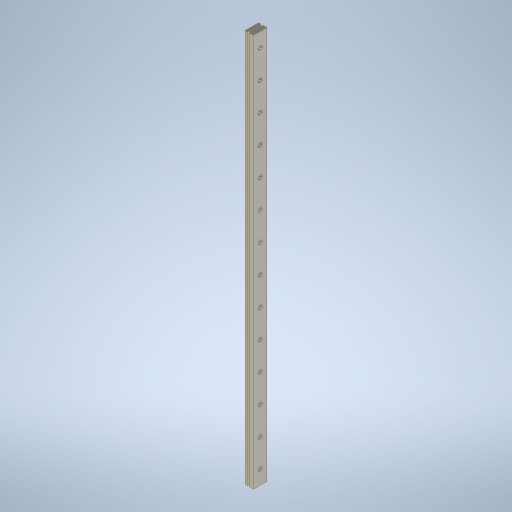
# Autodesk Inventor part: Trilho
Saved by Autodesk Inventor 2023 (Build 270158000, 158)
## iProperties
Created: 2023-03-17
Part Number: Trilho
Material: Aço inoxidável
Document SubType Name: Sheet Metal
Designer: Mateus
Density: 8 g/cm^3
Sheet Metal Rule: Default_mm
Appearance: Prata
Mass: 219.806 g
Surface Area: 172.742 cm^2
Volume: 27.4758 cm^3
Author: Mateus
Autodesk Inventor part; units mm, degrees
ref_plane "YZ Plane" through (0, 0, 0) normal (1, 0, 0) x (0, 1, 0)
ref_plane "XZ Plane" through (0, 0, 0) normal (0, 1, 0) x (-1, 0, 0)
ref_plane "XY Plane" through (0, 0, 0) normal (0, 0, 1) x (1, 0, 0)
sketch "Esboço1" plane through (0, 0, 0) normal (0, 1, 0) x (-1, 0, 0)
  line L0 (0, 0) -> (3.5, 0)
  line L1 (4, -2) -> (5, -2)
  line L2 (5.5, 0) -> (7.5, 0)
  line L3 (7.5, 0) -> (7.5, -12)
  line L4 (7.5, -12) -> (5.5, -12)
  line L5 (5, -10) -> (4, -10)
  line L6 (3.5, -12) -> (0, -12)
  line L7 (0, -12) -> (0, 0)
  line L8 (5.5, 0) -> (5, -2)
  line L9 (3.5, 0) -> (4, -2)
  line L10 (5, -10) -> (5.5, -12)
  line L11 (3.5, -12) -> (4, -10)
  dimension "d0" = 7.5
  dimension "d1" = 12
  dimension "d2" = 8
  dimension "d3" = 1
  dimension "d4" = 3.5
  dimension "d5" = 0.5
  constraints: 24 end point, 4 point on line, 3 equal length, 3 perpendicular, 1 horizontal, 1 parallel
  measures "d0" distance of L0.start L2.end
  measures "d1" distance of L6.end L0.start
  measures "d2" distance of L1.end L5.start
  measures "d3" distance of L1.start L1.end
  measures "d4" distance of L0.start L0.end
  measures "d5" horizontal distance of L2.start L1.end
extrude "Extrusão1" add sketch "Esboço1" along normal blind 350
sketch "Esboço2" plane through (-7.5, 0, -12) normal (-1, 0, 0) x (0, 0, 1)
  line L0 (0, 0) -> (12, 0) projected
  line L1 (12, 0) -> (12, 350) projected
  line L2 (0, 350) -> (12, 350) projected
  point P0 (6, 12.5)
  point P1 (6, 37.5)
  point P2 (6, 62.5)
  point P3 (6, 87.5)
  point P4 (6, 112.5)
  point P5 (6, 137.5)
  point P6 (6, 162.5)
  point P7 (6, 187.5)
  point P8 (6, 212.5)
  point P9 (6, 237.5)
  point P10 (6, 262.5)
  point P11 (6, 287.5)
  point P12 (6, 312.5)
  point P13 (6, 337.5)
  dimension "d8" = 25
  dimension "d9" = 12.5
  dimension "d10" = 12
  dimension "d11" = 6
  dimension "d12" = 6
  dimension "d13" = 25
  dimension "d14" = 25
  dimension "d15" = 25
  dimension "d16" = 25
  dimension "d17" = 25
  dimension "d18" = 25
  dimension "d19" = 25
  dimension "d20" = 25
  dimension "d21" = 25
  dimension "d22" = 25
  dimension "d23" = 25
  dimension "d24" = 25
  dimension "d25" = 12.5
  measures "d8" distance of point (6, 12.5) point (6, 37.5)
  measures "d9" distance from line of L0 point (6, 12.5)
  measures "d10" distance of L0.start L0.end
  measures "d11" distance from line of L1 point (6, 12.5)
  measures "d12" distance from line of L1 point (6, 287.5)
  measures "d13" distance of point (6, 62.5) point (6, 37.5)
  measures "d14" distance of point (6, 87.5) point (6, 62.5)
  measures "d15" distance of point (6, 112.5) point (6, 87.5)
  measures "d16" distance of point (6, 137.5) point (6, 112.5)
  measures "d17" distance of point (6, 137.5) point (6, 162.5)
  measures "d18" distance of point (6, 162.5) point (6, 187.5)
  measures "d19" distance of point (6, 187.5) point (6, 212.5)
  measures "d20" distance of point (6, 237.5) point (6, 212.5)
  measures "d21" distance of point (6, 237.5) point (6, 262.5)
  measures "d22" distance of point (6, 287.5) point (6, 262.5)
  measures "d23" distance of point (6, 287.5) point (6, 312.5)
  measures "d24" distance of point (6, 312.5) point (6, 337.5)
  measures "d25" distance from line of L2 point (6, 337.5)
hole "Furo1" at (-7.5, 12.5, -6) at (-7.5, 37.5, -6) at (-7.5, 62.5, -6) at (-7.5, 87.5, -6) at (-7.5, 112.5, -6) at (-7.5, 137.5, -6) at (-7.5, 162.5, -6) at (-7.5, 187.5, -6) at (-7.5, 212.5, -6) at (-7.5, 237.5, -6) at (-7.5, 262.5, -6) at (-7.5, 287.5, -6) at (-7.5, 312.5, -6) at (-7.5, 337.5, -6) direction (1, 0, 0) diameter 3.5 depth 7.5 counterbore diameter 6 counterbore depth 3.5
equation "\"d11\" = 0.5 * d10"
equation "\"d13\" = d8"
equation "\"d14\" = d13"
equation "\"d15\" = d13"
equation "\"d16\" = d14"
equation "\"d17\" = d16"
equation "\"d18\" = d17"
equation "\"d19\" = d17"
equation "\"d20\" = d18"
equation "\"d21\" = d19"
equation "\"d22\" = d20"
equation "\"d23\" = d21"
equation "\"d24\" = d22"
equation "\"d31\" = Espessura"
equation "\"Raio_vergadura\" = Espessura"
equation "\"Largura_alívio_de_vergadura\" = Espessura"
equation "\"Profundidade_alívio_de_vergadura\" = 0.5 * Espessura"
equation "\"Tamanho_alívio_de_dobra\" = 4 * Espessura"
equation "\"Remanescente_mínimo\" = 2 * Espessura"
equation "\"Raiodetransição\" = Raio_vergadura"
equation "\"Tamanho_de_raio_de_Jacobi\" = Raio_vergadura"
equation "\"TamanhoFolga\" = Espessura"
equation "\"Espessura\" = 0.5"
